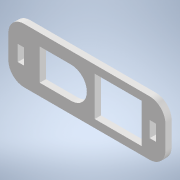
# Autodesk Inventor part: top2
Saved by Autodesk Inventor 2022 (Build 260153000, 153)
## iProperties
Created: 2025-06-24
Part Number: top2
Material: Типовые
Document SubType Name: Modeling
Designer: korsh524
Density: 1 g/cm^3
Appearance: По умолчанию
Author: korsh524
Autodesk Inventor part; units mm, degrees
ref_plane "YZ Plane" through (0, 0, 0) normal (1, 0, 0) x (0, 1, 0)
ref_plane "XZ Plane" through (0, 0, 0) normal (0, 1, 0) x (-1, 0, 0)
ref_plane "XY Plane" through (0, 0, 0) normal (0, 0, 1) x (1, 0, 0)
sketch "Эскиз1" plane through (0, 0, 0) normal (0, 0, 1) x (1, 0, 0)
  line L0 (-44, 4.453) -> (-40, 4.453) projected
  line L1 (-40, 4.453) -> (-40, -5.547) projected
  line L2 (-40, -5.547) -> (-44, -5.547) projected
  line L3 (-44, -5.547) -> (-44, 4.453) projected
  line L4 (-10, -10) -> (-30, -10) projected
  line L5 (-30, -10) -> (-30, 10) projected
  line L6 (-30, 10) -> (-10, 10) projected
  arc A0 (-10, -10) -> (-10, 10) centre (-10, 0) ccw projected
  line L7 (44, -5.547) -> (40, -5.547) projected
  line L8 (40, -5.547) -> (40, 4.453) projected
  line L9 (40, 4.453) -> (44, 4.453) projected
  line L10 (44, 4.453) -> (44, -5.547) projected
  arc A1 (-50, -7.5) -> (-40, -17.5) centre (-40, -7.5) ccw projected
  line L11 (40, -17.5) -> (-40, -17.5) projected
  arc A2 (40, -17.5) -> (50, -7.5) centre (40, -7.5) ccw projected
  line L12 (50, 7.5) -> (50, -7.5) projected
  arc A3 (50, 7.5) -> (40, 17.5) centre (40, 7.5) ccw projected
  line L13 (-40, 17.5) -> (40, 17.5) projected
  arc A4 (-40, 17.5) -> (-50, 7.5) centre (-40, 7.5) ccw projected
  line L14 (-50, -7.5) -> (-50, 7.5) projected
  line L15 (35, 12.5) -> (5, 12.5)
  line L16 (5, 12.5) -> (5, -12.5)
  line L17 (5, -12.5) -> (35, -12.5)
  line L18 (35, -12.5) -> (35, 12.5)
  point P0 (0, 0)
  dimension "d0" = 25
  dimension "d1" = 30
  dimension "d2" = 12.5
  dimension "d3" = 5
  constraints: 8 end point, 2 parallel, 1 horizontal, 1 perpendicular
  measures "d0" distance of L17.end L15.start
  measures "d1" distance of L15.start L15.end
  measures "d2" distance from line of point (0, 0) L17
  measures "d3" distance from line of L16 point (0, 0)
extrude "Выдавливание1" add sketch "Эскиз1" along normal blind 4
